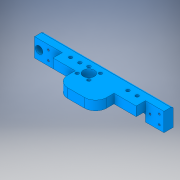
# Autodesk Inventor part: GripperM otorBlock
Saved by Autodesk Inventor 2019 (Build 230136000, 136)
## iProperties
Created: 2019-10-02
Part Number: GripperM otorBlock
Material: Generic
Document SubType Name: Modeling
Designer: james
Density: 1 g/cm^3
Appearance: Default(2)
Author: james
Autodesk Inventor part; units mm, degrees
ref_plane "YZ Plane" through (0, 0, 0) normal (1, 0, 0) x (0, 1, 0)
ref_plane "XZ Plane" through (0, 0, 0) normal (0, 1, 0) x (-1, 0, 0)
ref_plane "XY Plane" through (0, 0, 0) normal (0, 0, 1) x (1, 0, 0)
sketch "Sketch1" plane through (0, 0, 0) normal (1, 0, 0) x (0, 1, 0)
  line L0 (11.2985, 26.2091) -> (-1.4015, 26.2091)
  line L1 (-1.4015, 26.2091) -> (-1.4015, -24.5909)
  line L2 (-1.4015, -24.5909) -> (11.2985, -24.5909)
  line L3 (11.2985, -24.5909) -> (11.2985, 26.2091)
  point P0 (0, 0)
  dimension "d0" = 50.8
  dimension "d1" = 12.7
  constraints: 8 end point, 2 parallel, 1 horizontal, 1 perpendicular
  measures "d0" distance of L2.end L0.start
  measures "d1" distance of L0.start L0.end
extrude "Extrusion1" add sketch "Sketch1" along normal blind 165.1
sketch "Sketch2" plane through (0, 11.2985, 26.2091) normal (0, 1, 0) x (1, 0, 0)
  circle A0 centre (68.2625, 31.75) radius 12.7
  circle A1 centre (87.3125, 31.75) radius 12.7
  line L0 (0, 50.8) -> (0, 0) projected
  line L1 (0, 50.8) -> (165.1, 50.8) projected
  point P0 (0, 26.2091)
  point P1 (60.2615, 39.751)
  point P2 (76.2635, 39.751)
  point P3 (76.2635, 23.749)
  point P4 (60.2615, 23.749)
  dimension "d4" = 25.4
  dimension "d5" = 25.4
  dimension "d6" = 0
  dimension "d7" = 19.05
  dimension "d8" = 68.2625
  dimension "d9" = 19.05
  dimension "d46" = 0
  dimension "d47" = 0
  dimension "d48" = 0
  dimension "d49" = 0
  dimension "d50" = 16.002
  dimension "d51" = 16.002
  dimension "d52" = 8.001
  dimension "d53" = 8.001
  constraints: 2 centre point
  measures "d4" diameter of A0
  measures "d5" diameter of A1
  measures "d6" vertical distance of A0.centre A1.centre
  measures "d7" distance of A0.centre A1.centre
  measures "d8" distance from line of L0 A0.centre
  measures "d9" distance from line of L1 A0.centre
  measures "d46" horizontal distance of point (60.262, 23.749) point (60.262, 39.751)
  measures "d47" horizontal distance of point (76.264, 39.751) point (76.264, 23.749)
  measures "d48" vertical distance of point (60.262, 23.749) point (76.264, 23.749)
  measures "d49" vertical distance of point (60.262, 39.751) point (76.264, 39.751)
  measures "d50" distance of point (76.264, 39.751) point (60.262, 39.751)
  measures "d51" distance of point (60.262, 23.749) point (60.262, 39.751)
  measures "d52" horizontal distance of point (60.262, 39.751) A0.centre
  measures "d53" horizontal distance of A0.centre point (60.262, 23.749)
sketch "Sketch8" plane through (0, 11.2985, 26.2091) normal (0, 1, 0) x (1, 0, 0)
  line L0 (-37.599, -14.8006) -> (55.88, -14.8006)
  line L1 (55.88, -14.8006) -> (55.88, 38.1)
  line L2 (55.88, 38.1) -> (-37.599, 38.1)
  line L3 (-37.599, 38.1) -> (-37.599, -14.8006)
  line L4 (109.22, -16.386) -> (193.9952, -16.386)
  line L5 (193.9952, -16.386) -> (193.9952, 38.1)
  line L6 (193.9952, 38.1) -> (109.22, 38.1)
  line L7 (109.22, 38.1) -> (109.22, -16.386)
  line L8 (0, 50.8) -> (165.1, 50.8) projected
  line L9 (0, 50.8) -> (0, 0) projected
  line L10 (165.1, 50.8) -> (165.1, 0) projected
  point P0 (0, 26.2091)
  dimension "d36" = 12.7
  dimension "d37" = 55.88
  dimension "d38" = 12.7
  dimension "d39" = 55.88
  constraints: 16 end point, 4 parallel, 2 horizontal, 2 perpendicular
  measures "d36" distance between parallel lines of L2 L8
  measures "d37" distance between parallel lines of L9 L1
  measures "d38" distance between parallel lines of L8 L6
  measures "d39" distance between parallel lines of L10 L7
extrude "Extrusion8" cut sketch "Sketch8" against normal blind 76.2
fillet "Fillet1" radius 15.24 1 edges at (109.22, 4.9485, 26.2091)
fillet "Fillet2" radius 15.24 1 edges at (55.88, 4.9485, 26.2091)
hole "Hole1" at (60.2615, 11.2985, -13.5419) at (76.2635, 11.2985, -13.5419) at (76.2635, 11.2985, 2.4601) at (60.2615, 11.2985, 2.4601) direction (0, -1, 0) diameter 4.4958 end through all clearance for "Flat Head Machine Screw" size "M4" standard "Ansi Metric M Profile"
sketch "Sketch10" plane through (0, 11.2985, -24.5909) normal (0, 1, 0) x (1, 0, 0)
  circle A0 centre (76.2635, -27.051) radius 2.2479 projected
  circle A1 centre (60.2615, -11.049) radius 2.2479 projected
  circle A2 centre (60.2615, -27.051) radius 2.2479 projected
  circle A3 centre (76.2635, -11.049) radius 2.2479 projected
  line L0 (76.2635, -11.049) -> (60.2615, -27.051)
  line L1 (60.2615, -11.049) -> (76.2635, -27.051)
  point P0 (0, -24.5909)
  point P1 (68.2625, -19.05)
  dimension "d61" = 8.001
  dimension "d62" = 8.001
  constraints: 4 end point
  measures "d61" horizontal distance of point (68.263, -19.05) L1.start
  measures "d62" horizontal distance of point (68.263, -19.05) L0.start
hole "Hole2" at (68.2625, 11.2985, -5.5409) direction (0, -1, 0) diameter 15.24 end through all
sketch "Sketch11" plane through (0, 11.2985, -11.8909) normal (0, 0, 1) x (1, 0, 0)
  line L0 (55.88, 0) -> (0, 0)
  line L1 (0, 0) -> (0, -12.7)
  line L2 (0, -12.7) -> (55.88, -12.7)
  line L3 (55.88, -12.7) -> (55.88, 0)
  line L4 (0, -12.7) -> (0, 0) projected
  line L5 (55.88, 0) -> (55.88, -12.7) projected
  line L6 (0, 0) -> (55.88, 0) projected
  line L7 (55.88, -12.7) -> (0, -12.7) projected
  point P0 (0, -11.2985)
  dimension "d70" = 0
  dimension "d71" = 0
  dimension "d72" = 0
  dimension "d73" = 0
  constraints: 8 end point, 2 parallel, 1 horizontal, 1 perpendicular
  measures "d70" distance between parallel lines of L4 L1
  measures "d71" distance between parallel lines of L5 L3
  measures "d72" distance between parallel lines of L6 L0
  measures "d73" distance between parallel lines of L7 L2
extrude "Extrusion9" add sketch "Sketch11" along normal blind 12.7
sketch "Sketch12" plane through (109.22, 11.2985, -11.8909) normal (0, 0, 1) x (1, 0, 0)
  line L0 (0, 0) -> (55.88, 0)
  line L1 (55.88, 0) -> (55.88, -12.7)
  line L2 (55.88, -12.7) -> (0, -12.7)
  line L3 (0, -12.7) -> (0, 0)
  line L4 (55.88, 0) -> (55.88, -12.7) projected
  line L5 (0, 0) -> (55.88, 0) projected
  line L6 (55.88, -12.7) -> (0, -12.7) projected
  line L7 (0, -12.7) -> (0, 0) projected
  point P0 (-109.22, -11.2985)
  dimension "d76" = 0
  dimension "d77" = 0
  dimension "d78" = 0
  dimension "d79" = 0
  constraints: 8 end point, 2 parallel, 1 horizontal, 1 perpendicular
  measures "d76" distance between parallel lines of L4 L1
  measures "d77" distance between parallel lines of L5 L0
  measures "d78" distance between parallel lines of L6 L2
  measures "d79" distance between parallel lines of L7 L3
extrude "Extrusion10" add sketch "Sketch12" along normal blind 12.7
sketch "Sketch13" plane through (0, 11.2985, -24.5909) normal (0, 1, 0) x (1, 0, 0)
  line L0 (55.88, -25.4) -> (55.88, -35.56) projected
  line L1 (0, 0) -> (165.1, 0) projected
  line L2 (109.22, -35.56) -> (109.22, -25.4) projected
  point P0 (0, -24.5909)
  point P1 (49.53, -12.7)
  point P2 (36.83, -12.7)
  point P3 (115.57, -12.7)
  point P4 (128.27, -12.7)
  dimension "d82" = 19.05
  dimension "d83" = 6.35
  dimension "d84" = 12.7
  dimension "d85" = 12.7
  dimension "d86" = 6.35
  dimension "d87" = 19.05
  dimension "d88" = 12.7
  dimension "d89" = 12.7
  measures "d82" distance from line of L0 point (36.83, -12.7)
  measures "d83" distance from line of L0 point (49.53, -12.7)
  measures "d84" distance from line of L1 point (49.53, -12.7)
  measures "d85" distance from line of L1 point (36.83, -12.7)
  measures "d86" distance from line of L2 point (115.57, -12.7)
  measures "d87" distance from line of L2 point (128.27, -12.7)
  measures "d88" distance from line of L1 point (115.57, -12.7)
  measures "d89" distance from line of L1 point (128.27, -12.7)
hole "Hole3" at (49.53, 11.2985, -11.8909) at (36.83, 11.2985, -11.8909) at (115.57, 11.2985, -11.8909) at (128.27, 11.2985, -11.8909) direction (0, -1, 0) diameter 4.4958 depth 25.4 tip angle 118.188 clearance for "Flat Head Machine Screw (82)" size "#8" standard "Ansi Unified Screw Threads"
sketch "Sketch14" plane through (0, 11.2985, -24.5909) normal (0, 1, 0) x (1, 0, 0)
  line L0 (0, 0) -> (25.4, 0)
  line L1 (25.4, 0) -> (25.4, -25.4)
  line L2 (25.4, -25.4) -> (0, -25.4)
  line L3 (0, -25.4) -> (0, 0)
  line L4 (165.1, 0) -> (139.7, 0)
  line L5 (139.7, 0) -> (139.7, -25.4)
  line L6 (139.7, -25.4) -> (165.1, -25.4)
  line L7 (165.1, -25.4) -> (165.1, 0)
  line L8 (0, 0) -> (165.1, 0) projected
  line L9 (165.1, 0) -> (165.1, -25.4) projected
  line L10 (165.1, -25.4) -> (109.22, -25.4) projected
  line L11 (0, 0) -> (0, -25.4) projected
  line L12 (55.88, -25.4) -> (0, -25.4) projected
  point P0 (0, -24.5909)
  dimension "d97" = 0
  dimension "d98" = 25.4
  dimension "d99" = 0
  dimension "d100" = 0
  dimension "d101" = 25.4
  dimension "d102" = 0
  dimension "d103" = 0
  dimension "d104" = 0
  constraints: 16 end point, 4 parallel, 2 horizontal, 2 perpendicular
  measures "d97" distance between parallel lines of L8 L4
  measures "d98" distance between parallel lines of L7 L5
  measures "d99" distance between parallel lines of L9 L7
  measures "d100" distance between parallel lines of L10 L6
  measures "d101" distance of L1.end L2.end
  measures "d102" distance between parallel lines of L11 L3
  measures "d103" distance between parallel lines of L12 L2
  measures "d104" distance between parallel lines of L8 L0
extrude "Extrusion11" add sketch "Sketch14" against normal blind 25.4
sketch "Sketch16" plane through (0, -14.1015, -24.5909) normal (0, -1, 0) x (1, 0, 0)
  line L0 (-15.071, 42.5671) -> (25.4, 42.5671)
  line L1 (25.4, 42.5671) -> (25.4, 12.7)
  line L2 (25.4, 12.7) -> (-15.071, 12.7)
  line L3 (-15.071, 12.7) -> (-15.071, 42.5671)
  line L4 (139.7, 42.5671) -> (181.0335, 42.5671)
  line L5 (181.0335, 42.5671) -> (181.0335, 12.7)
  line L6 (181.0335, 12.7) -> (139.7, 12.7)
  line L7 (139.7, 12.7) -> (139.7, 42.5671)
  line L8 (165.1, 25.4) -> (139.7, 25.4) projected
  line L9 (139.7, 25.4) -> (139.7, 0) projected
  line L10 (25.4, 0) -> (25.4, 25.4) projected
  line L11 (25.4, 25.4) -> (0, 25.4) projected
  point P0 (0, 24.5909)
  dimension "d112" = 12.7
  dimension "d113" = 0
  dimension "d114" = 0
  dimension "d115" = 12.7
  constraints: 16 end point, 4 parallel, 2 horizontal, 2 perpendicular, 1 point on line
  measures "d112" distance between parallel lines of L6 L8
  measures "d113" distance between parallel lines of L9 L7
  measures "d114" distance between parallel lines of L10 L1
  measures "d115" distance between parallel lines of L2 L11
extrude "Extrusion13" cut sketch "Sketch16" against normal blind 50.8
sketch "Sketch17" plane through (0, -14.1015, -11.8909) normal (0, 0, 1) x (1, 0, 0)
  line L0 (0, 0) -> (0, 25.4) projected
  line L1 (0, 25.4) -> (25.4, 25.4) projected
  line L2 (25.4, 0) -> (0, 0) projected
  line L3 (165.1, 25.4) -> (165.1, 0) projected
  line L4 (139.7, 25.4) -> (165.1, 25.4) projected
  line L5 (165.1, 0) -> (139.7, 0) projected
  point P0 (0, 14.1015)
  point P1 (6.35, 19.05)
  point P2 (6.35, 6.35)
  point P3 (19.05, 12.7)
  point P4 (146.05, 12.7)
  point P5 (158.75, 19.05)
  point P6 (158.75, 6.35)
  dimension "d118" = 6.35
  dimension "d119" = 6.35
  dimension "d120" = 6.35
  dimension "d121" = 6.35
  dimension "d122" = 19.05
  dimension "d123" = 12.7
  dimension "d124" = 19.05
  dimension "d125" = 12.7
  dimension "d126" = 6.35
  dimension "d127" = 6.35
  dimension "d128" = 6.35
  dimension "d129" = 6.35
  measures "d118" distance from line of L0 point (6.35, 19.05)
  measures "d119" distance from line of L1 point (6.35, 19.05)
  measures "d120" distance from line of L0 point (6.35, 6.35)
  measures "d121" distance from line of L2 point (6.35, 6.35)
  measures "d122" distance from line of L0 point (19.05, 12.7)
  measures "d123" distance from line of L2 point (19.05, 12.7)
  measures "d124" distance from line of L3 point (146.05, 12.7)
  measures "d125" distance from line of L4 point (146.05, 12.7)
  measures "d126" distance from line of L3 point (158.75, 19.05)
  measures "d127" distance from line of L3 point (158.75, 6.35)
  measures "d128" distance from line of L5 point (158.75, 6.35)
  measures "d129" distance from line of L4 point (158.75, 19.05)
hole "Hole4" at (6.35, 4.9485, -11.8909) at (6.35, -7.7515, -11.8909) at (19.05, -1.4015, -11.8909) at (146.05, -1.4015, -11.8909) at (158.75, 4.9485, -11.8909) at (158.75, -7.7515, -11.8909) direction (0, 0, -1) diameter 2.6416 depth 10.9728 tip angle 118.188 thread size "6-32 UNC" class "2B" standard "ANSI Unified Screw Threads"
sketch "Sketch18" plane through (71.12, -1.4015, 26.2091) normal (0, -1, 0) x (1, 0, 0)
  line L0 (-45.72, -45.72) -> (68.58, -45.72)
  line L1 (68.58, -45.72) -> (68.58, -50.8)
  line L2 (68.58, -50.8) -> (-45.72, -50.8)
  line L3 (-45.72, -50.8) -> (-45.72, -45.72)
  line L4 (-45.72, -50.8) -> (68.58, -50.8) projected
  line L5 (68.58, -38.1) -> (68.58, -50.8) projected
  line L6 (-45.72, -50.8) -> (-45.72, -38.1) projected
  point P0 (-71.12, -26.2091)
  dimension "d137" = 0
  dimension "d138" = 0
  dimension "d139" = 5.08
  dimension "d140" = 0
  constraints: 8 end point, 2 parallel, 1 horizontal, 1 perpendicular
  measures "d137" distance between parallel lines of L4 L2
  measures "d138" distance between parallel lines of L5 L1
  measures "d139" distance between parallel lines of L2 L0
  measures "d140" distance between parallel lines of L6 L3
extrude "Extrusion14" add sketch "Sketch18" along normal blind 12.7
sketch "Sketch19" plane through (165.1, 11.2985, -24.5909) normal (0, 0, -1) x (-1, 0, 0)
  line L0 (82.55, -51.592) -> (82.55, 23.9487)
  line L1 (165.1, 0) -> (165.1, -25.4) projected
  line L2 (0, 0) -> (0, -25.4) projected
  arc A0 (134.9134, -25.4) -> (30.1866, -25.4) centre (82.55, -127) ccw
  line L3 (165.1, -25.4) -> (0, -25.4) projected
  line L4 (134.9134, -25.4) -> (30.1866, -25.4)
  point P0 (165.1, -11.2985)
  dimension "d143" = 82.55
  dimension "d144" = 82.55
  dimension "d145" = 0
  dimension "d146" = 101.6
  dimension "d147" = 228.6
  constraints: 4 end point, 2 point on circle, 1 centre point, 1 vertical
  measures "d143" distance between parallel lines of L1 L0
  measures "d144" distance between parallel lines of L2 L0
  measures "d145" distance from line of L0 A0.centre
  measures "d146" distance from line of L3 A0.centre
  measures "d147" diameter of A0
extrude "Extrusion15" cut sketch "Sketch19" against normal blind 6.35
sketch "Sketch20" plane through (0, 0, 0) normal (-1, 0, 0) x (0, 0, 1)
  line L0 (-24.5909, 11.2985) -> (-24.5909, -14.1015) projected
  line L1 (-11.8909, -14.1015) -> (-24.5909, -14.1015) projected
  line L2 (-11.8909, -14.1015) -> (-11.8909, 11.2985) projected
  line L3 (-24.5909, 11.2985) -> (-11.8909, 11.2985) projected
  line L4 (-11.8909, -14.1015) -> (-11.8909, -1.4015) projected
  line L5 (-11.8909, -14.1015) -> (-24.5909, -14.1015)
  line L6 (-24.5909, -14.1015) -> (-24.5909, 11.2985)
  line L7 (-24.5909, 11.2985) -> (-11.8909, 11.2985)
  line L8 (-11.8909, 11.2985) -> (-11.8909, -14.1015)
  point P0 (0, 0)
  constraints: 8 end point, 2 parallel, 1 horizontal, 1 perpendicular
extrude "Extrusion16" add sketch "Sketch20" along normal blind 12.7
sketch "Sketch21" plane through (25.4, -14.1015, -11.8909) normal (0, 0, 1) x (1, 0, 0)
  line L0 (0, 0) -> (-38.1, 0) projected
  line L1 (-38.1, 0) -> (-38.1, 25.4) projected
  point P0 (-25.4, 14.1015)
  point P1 (-31.75, 12.7)
  dimension "d152" = 12.7
  dimension "d153" = 6.35
  measures "d152" distance from line of L0 point (-31.75, 12.7)
  measures "d153" distance from line of L1 point (-31.75, 12.7)
hole "Hole5" at (-6.35, -1.4015, -11.8909) direction (0, 0, -1) diameter 10.16 depth 12.2936 tip angle 118.188
fillet "Fillet3" radius 3.175 1 edges at (76.2, 11.2985, -24.5909)
body "Solid1"
